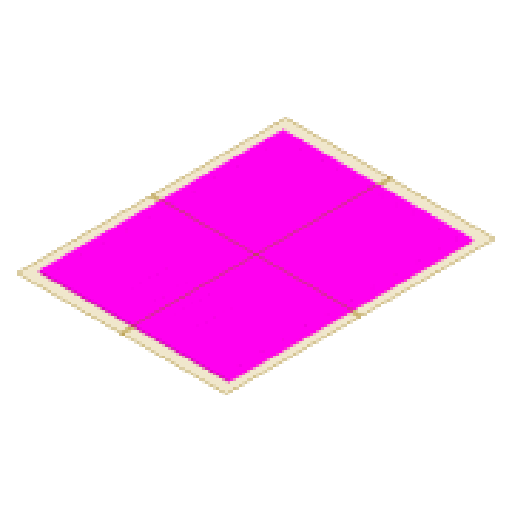
# Autodesk Inventor part: Фанера_крышки
Saved by Autodesk Inventor 2023.2 (Build 272271030, 271C)
## iProperties
Created: 2025-05-05
Part Number: Фанера_крышки
Material: Типовые
Document SubType Name: Modeling
Designer: Олег Коноваленко
Density: 1 g/cm^3
Appearance: Пурпурный
Author: Олег Коноваленко
Autodesk Inventor part; units mm, degrees
sketch "Эскиз1" plane through (0, 0, 0) normal (0, 1, 0) x (-1, 0, 0)
  line L0 (170, -218.5) -> (-170, -218.5)
  line L1 (-170, -218.5) -> (-170, 218.5)
  line L2 (-170, 218.5) -> (170, 218.5)
  line L3 (170, 218.5) -> (170, -218.5)
  line L4 (170, -218.5) -> (-170, 218.5) construction
  line L5 (-170, -218.5) -> (170, 218.5) construction
  point P0 (0, 0)
  point P1 (0, 0)
  dimension "d0" = 340
  dimension "d1" = 437
  constraints: 12 end point, 2 parallel, 1 coincident, 1 horizontal, 1 midpoint, 1 perpendicular
  measures "d0" distance between parallel lines of L1 L3
  measures "d1" distance between parallel lines of L2 L0
extrude "Выдавливание1" add sketch "Эскиз1" along normal mid plane 4
sketch "Эскиз3" plane through (0, 2, 0) normal (0, 1, 0) x (1, 0, 0)
  circle A0 centre (-155, -198.5) radius 2 projected
  circle A1 centre (-155, -158.5) radius 2 projected
  circle A2 centre (-155, -118.5) radius 2 projected
  circle A3 centre (-155, -78.5) radius 2 projected
  circle A4 centre (-155, -38.5) radius 2 projected
  circle A5 centre (-155, 1.5) radius 2 projected
  circle A6 centre (-155, 41.5) radius 2 projected
  circle A7 centre (-155, 81.5) radius 2 projected
  circle A8 centre (-155, 121.5) radius 2 projected
  circle A9 centre (-155, 173.5) radius 2 projected
  circle A10 centre (-155, 203.5) radius 2 projected
  circle A11 centre (-125, 203.5) radius 2 projected
  circle A12 centre (-86, 203.5) radius 2 projected
  circle A13 centre (-59, 203.5) radius 2 projected
  circle A14 centre (-32, 203.5) radius 2 projected
  circle A15 centre (-5, 203.5) radius 2 projected
  circle A16 centre (22, 203.5) radius 2 projected
  circle A17 centre (49, 203.5) radius 2 projected
  circle A18 centre (76, 203.5) radius 2 projected
  circle A19 centre (125, 203.5) radius 2 projected
  circle A20 centre (155, 203.5) radius 2 projected
  circle A21 centre (155, 173.5) radius 2 projected
  circle A22 centre (155, 133.5) radius 2 projected
  circle A23 centre (155, 93.5) radius 2 projected
  circle A24 centre (155, 53.5) radius 2 projected
  circle A25 centre (155, 13.5) radius 2 projected
  circle A26 centre (155, -26.5) radius 2 projected
  circle A27 centre (155, -66.5) radius 2 projected
  circle A28 centre (155, -106.5) radius 2 projected
  circle A29 centre (155, -146.5) radius 2 projected
  circle A30 centre (155, -186.5) radius 2 projected
  circle A31 centre (60, -103.5008) radius 1.15 projected
  circle A32 centre (60, -118.5008) radius 1.15 projected
  circle A33 centre (60, -133.5008) radius 1.15 projected
  circle A34 centre (60, -148.5008) radius 1.15 projected
  circle A35 centre (60, -163.5008) radius 1.15 projected
  circle A36 centre (20, -148.5008) radius 1.15 projected
  circle A37 centre (20, -133.5008) radius 1.15 projected
  circle A38 centre (20, -118.5008) radius 1.15 projected
  circle A39 centre (20, -103.5008) radius 1.15 projected
  circle A40 centre (-20, -148.5008) radius 1.15 projected
  circle A41 centre (-20, -133.5008) radius 1.15 projected
  circle A42 centre (-20, -118.5008) radius 1.15 projected
  circle A43 centre (-20, -103.5008) radius 1.15 projected
  circle A44 centre (-60, -148.5008) radius 1.15 projected
  circle A45 centre (-60, -133.5008) radius 1.15 projected
  circle A46 centre (-60, -118.5008) radius 1.15 projected
  circle A47 centre (-60, -103.5008) radius 1.15 projected
  circle A48 centre (20, -163.5008) radius 1.15 projected
  circle A49 centre (-60, -163.5008) radius 1.15 projected
  circle A50 centre (-20, -163.5008) radius 1.15 projected
  point P0 (0, 0)
extrude "Выдавливание3" cut sketch "Эскиз3" against normal up to surface (4 mm away) contours A0 | A1 | A2 | A3 | A4 | A5 | A6 | A7 | A8 | A9 | A11 | A12 | A13 | A14 | A15 | A16 | A17 | A18 | A19 | A20 | A21 | A22 | A23 | A24 | A25 | A26 | A27 | A28 | A29 | A30 | A31 | A32 | A33 | A34 | A35 | A36 | A37 | A38 | A39 | A40 | A41 | A42 | A43 | A44 | A45 | A46 | A47 | A48 | A49 | A50
